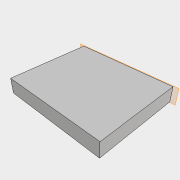
# Autodesk Inventor part: ЛЦМК.00002.00.00.00.00.21 Контакты
Saved by Autodesk Inventor 2021.2 (Build 252289000, 289)
## iProperties
Created: 2025-11-19
Part Number: ЛЦМК.00002.00.00.00.00.21 Контакты
Material: Типовые
Document SubType Name: Modeling
Designer: Захаров
Density: 1 g/cm^3
Appearance: По умолчанию
Author: Захаров
Autodesk Inventor part; units mm, degrees
ref_plane "YZ Plane" through (0, 0, 0) normal (1, 0, 0) x (0, 1, 0)
ref_plane "XZ Plane" through (0, 0, 0) normal (0, 1, 0) x (-1, 0, 0)
ref_plane "XY Plane" through (0, 0, 0) normal (0, 0, 1) x (1, 0, 0)
ref_plane "РабПлоскость1" through (0, 0, 0) normal (0, 0, 1) x (1, 0, 0)
sketch "Эскиз1" plane through (0, 0, 0) normal (0, 0, 1) x (1, 0, 0)
  line L0 (-10.35, -0.8) -> (-11.95, -0.8) projected
  line L1 (-11.95, -0.8) -> (-11.95, 0.8) projected
  line L2 (-11.95, 0.8) -> (-10.35, 0.8) projected
  line L3 (-10.35, 0.8) -> (-10.35, -0.8) projected
  line L4 (-3.15, -0.8) -> (-4.75, -0.8) projected
  line L5 (-4.75, -0.8) -> (-4.75, 0.8) projected
  line L6 (-4.75, 0.8) -> (-3.15, 0.8) projected
  line L7 (-3.15, 0.8) -> (-3.15, -0.8) projected
  line L8 (-5.55, -0.8) -> (-7.15, -0.8) projected
  line L9 (-7.15, -0.8) -> (-7.15, 0.8) projected
  line L10 (-7.15, 0.8) -> (-5.55, 0.8) projected
  line L11 (-5.55, 0.8) -> (-5.55, -0.8) projected
  line L12 (-12.75, -0.8) -> (-14.35, -0.8) projected
  line L13 (-14.35, -0.8) -> (-14.35, 0.8) projected
  line L14 (-14.35, 0.8) -> (-12.75, 0.8) projected
  line L15 (-12.75, 0.8) -> (-12.75, -0.8) projected
  line L16 (-15.15, -0.8) -> (-16.75, -0.8) projected
  line L17 (-16.75, -0.8) -> (-16.75, 0.8) projected
  line L18 (-16.75, 0.8) -> (-15.15, 0.8) projected
  line L19 (-15.15, 0.8) -> (-15.15, -0.8) projected
  line L20 (-7.95, -0.8) -> (-9.55, -0.8) projected
  line L21 (-9.55, -0.8) -> (-9.55, 0.8) projected
  line L22 (-9.55, 0.8) -> (-7.95, 0.8) projected
  line L23 (-7.95, 0.8) -> (-7.95, -0.8) projected
  line L24 (-0.75, -0.8) -> (-2.35, -0.8) projected
  line L25 (-2.35, -0.8) -> (-2.35, 0.8) projected
  line L26 (-2.35, 0.8) -> (-0.75, 0.8) projected
  line L27 (-0.75, 0.8) -> (-0.75, -0.8) projected
  line L28 (-17.5, -1.3) -> (-17.5, 1.3) projected
  line L29 (0, -1.3) -> (-17.5, -1.3) projected
  line L30 (0, -1.3) -> (0, 1.3) projected
  line L31 (-17.5, 1.3) -> (0, 1.3) projected
  point P0 (0, 0)
extrude "Выдавливание1" add sketch "Эскиз1" along normal blind 14.5 contours L0 L1 L2 L3 | L4 L5 L6 L7 | L8 L9 L10 L11 | L12 L13 L14 L15 | L16 L17 L18 L19 | L20 L21 L22 L23 | L24 L25 L26 L27 | L28 L31 L30 L29
